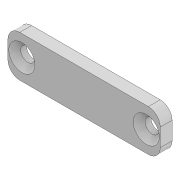
# Autodesk Inventor part: Пластина
Saved by Autodesk Inventor 2021 (Build 250183000, 183)
## iProperties
Created: 2023-02-18
Part Number: Пластина
Material: Типовые
Document SubType Name: Modeling
Designer: Tasya
Density: 1 g/cm^3
Appearance: По умолчанию
Author: Tasya
Autodesk Inventor part; units mm, degrees
ref_plane "YZ Plane" through (0, 0, 0) normal (1, 0, 0) x (0, 1, 0)
ref_plane "XZ Plane" through (0, 0, 0) normal (0, 1, 0) x (-1, 0, 0)
ref_plane "РабПлоскость1" through (0, 0, 0) normal (0, 0, 1) x (1, 0, 0)
sketch "Эскиз1" plane through (0, 0, 0) normal (0, 0, 1) x (1, 0, 0)
  circle A0 centre (16.2144, 37.6051) radius 1.45 construction
  arc A1 (18.5644, 39.1051) -> (16.5644, 41.1051) centre (16.5644, 39.1051) ccw projected
  line L0 (16.5644, 41.1051) -> (-5.1356, 41.1051) projected
  arc A2 (-5.1356, 41.1051) -> (-7.1356, 39.1051) centre (-5.1356, 39.1051) ccw projected
  line L1 (-7.1356, 39.1051) -> (-7.1356, 36.1051) projected
  arc A3 (-7.1356, 36.1051) -> (-5.1356, 34.1051) centre (-5.1356, 36.1051) ccw projected
  line L2 (-5.1356, 34.1051) -> (16.5644, 34.1051) projected
  arc A4 (16.5644, 34.1051) -> (18.5644, 36.1051) centre (16.5644, 36.1051) ccw projected
  line L3 (18.5644, 36.1051) -> (18.5644, 39.1051) projected
  circle A5 centre (-4.7856, 37.6051) radius 1.45 construction
  point P0 (0, 0)
extrude "Выдавливание1" add sketch "Эскиз1" along normal blind 2
sketch "Эскиз2" plane through (0, 0, 2) normal (0, 0, 1) x (1, 0, 0)
  circle A0 centre (-4.7856, 37.6051) radius 1.25 projected
  circle A1 centre (16.2144, 37.6051) radius 1.25 projected
  point P0 (0, 0)
  constraints: 2 coincident
hole "Отверстие1" at (16.2144, 37.6051, 2) at (-4.7856, 37.6051, 2) direction (0, 0, -1) diameter 2.4 depth 4 countersink diameter 4.4 countersink angle 90 clearance for "с потайной головкой ГОСТ 12876-67" size "M2" standard "ГОСТ"
